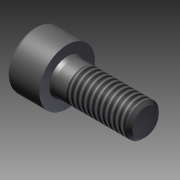
# Autodesk Inventor part: Zylinderschraube ISO 4762 - screw - M5x12-screw
Saved by Autodesk Inventor 2011 SP1 (Build 150282100, 282)
## iProperties
Created: 2016-04-05
Part Number: Zylinderschraube ISO 4762 - screw - M5x12-screw
Catalog Web Link: www.cadenas.de
Description: ISO 4762 - screw-Hexagon socket head cap screw
Vendor: MISUMI
Document SubType Name: Modeling
Designer: psAdmin
Manufacturer: MISUMI
Mass: 0.469354 g
Surface Area: 4.67275 cm^2
Volume: 0.469354 cm^3
Density: 1 g/cm^3
Category: PARTsolutions
Company: MISUMI
Title: Zylinderschraube ISO 4762 - screw - M5x12-screw
Author: Cadenas PARTsolutions
Comments: Hexagon socket head cap screw
PSOL_IDENT_0: {$CADENAS_DATA\23d-libs\misumi\metric\02_shaft_supports\screw.prj},247 {VTYP=3D},{NB=Zylinderschraub
PSOL_IDENT_1: e ISO 4762 - screw - M5x12-screw},{LINA=Zylinderschraube ISO 4762 - screw - M5x12-screw},{NN=ISO 476
PSOL_IDENT_2: 2 - screw},{DATE=22.04.2015 10:30:10},{GEOMDATE=13.12.2010 08:58:00},{VERSION=},{LINEID=490},{LINESU
PSOL_IDENT_3: BID=-1},{WBVAR=}  {NB=Zylinderschraube ISO 4762 - screw - M5x12-screw},{LINA=Zylinderschraube ISO 47
PSOL_IDENT_4: 62 - screw - M5x12-screw},{KT=DUMMY},{IDNR=},{D=5.000},{D3=4.019},{P=0.800},{L=12.000},{S=4.000},{HM=
PSOL_IDENT_5: 12.000},{DK=8.500},{DA=5.700},{DS=5.000},{E=4.580},{K=5.000},{R=0.200},{T=2.500},{V=0.500},{DW=8.030
PSOL_IDENT_6: },{W=1.900},{LF=0.600},{LG=2.400},{FORM=1.000},{NENN=M5x12-screw}
NN: ISO 4762 - screw
NT: Hexagon socket head cap screw
NB: Zylinderschraube ISO 4762 - screw - M5x12-screw
NBSYN: Zylinderschraube ISO 4762 - screw - $NENN.
LINA: Zylinderschraube ISO 4762 - screw - M5x12-screw
ROWDESC: M5x12-screw
D: 5.000
D3: 4.019
P: 0.800
L: 12.000
S: 4.000
HM: 12.000
DK: 8.500
DA: 5.700
DS: 5.000
E: 4.580
K: 5.000
R: 0.200
T: 2.500
V: 0.500
DW: 8.030
W: 1.900
LF: 0.600
LG: 2.400
FORM: 1.000
SUPPLIER: MISUMI
ARTICLENO: Zylinderschraube ISO 4762 - screw - M5x12-screw
BOMINFO: Zylinderschraube ISO 4762 - screw - M5x12-screw
CREATOR: CADENAS GmbH
Autodesk Inventor part; units mm, degrees
sketch "Skizze_2" plane through (0, 0, 0) normal (0, 0, 1) x (1, 0, 0)
  line L0 (12, 0) -> (-8, 0)
  line L1 (-0.7453, 0) -> (-1.9, 2)
  line L2 (-1.9, 2) -> (-5, 2)
  line L3 (-5, 2) -> (-5, 3.75)
  arc A0 (-4.5, 4.25) -> (-5, 3.75) centre (-4.5, 3.75) ccw
  line L4 (-4.5, 4.25) -> (0, 4.25)
  line L5 (0, 4.25) -> (0, 2.7114)
  line L6 (0, 2.7114) -> (0.5637, 2.5)
  line L7 (0.5637, 2.5) -> (11.5095, 2.5)
  line L8 (11.5095, 2.5) -> (12, 2.0095)
  line L9 (12, 2.0095) -> (12, 0)
  line L10 (12, 0) -> (-0.7453, 0)
  constraints: 22 end point, 2 point on circle, 1 centre point
revolve "Revolution1" add sketch "Skizze_2" angle 360 about axis through (12, 0, 0) along (1, 0, 0)
thread "Thread1" size "M5x0.8" class "6g" standard "ISO Metric profile" length 9.1095
sketch "Skizze_1" plane through (-1.9, 0, 0) normal (1, 0, 0) x (0, 0, -1)
  line L0 (-2, 1.1547) -> (-2, -1.1547)
  line L1 (-2, -1.1547) -> (0, -2.3094)
  line L2 (0, -2.3094) -> (2, -1.1547)
  line L3 (2, -1.1547) -> (2, 1.1547)
  line L4 (2, 1.1547) -> (0, 2.3094)
  line L5 (0, 2.3094) -> (-2, 1.1547)
  constraints: 12 end point
extrude "Extrusion1" cut sketch "Skizze_1" against normal blind 5
ref_plane "IP1_XY" through (0, 0, 0) normal (1, 0, 0) x (0, 0, -1)
ref_plane "IP1_YZ" through (0, 0, 0) normal (0, 0, -1) x (0, 1, 0)
ref_plane "IP1_ZX" through (0, 0, 0) normal (0, 1, 0) x (1, 0, 0)
ref_plane "IP2_XY" through (-5, 0, 0) normal (1, 0, 0) x (0, 0, -1)
ref_plane "IP2_YZ" through (-5, 0, 0) normal (0, 0, -1) x (0, 1, 0)
ref_plane "IP2_ZX" through (-5, 0, 0) normal (0, 1, 0) x (1, 0, 0)
ref_plane "IP3_XY" through (12, 0, 0) normal (1, 0, 0) x (0, 0, -1)
ref_plane "IP3_YZ" through (12, 0, 0) normal (0, 0, -1) x (0, 1, 0)
ref_plane "IP3_ZX" through (12, 0, 0) normal (0, 1, 0) x (1, 0, 0)
ref_plane "IP4_XY" through (0, 0, 0) normal (1, 0, 0) x (0, 0, -1)
ref_plane "IP4_YZ" through (0, 0, 0) normal (0, 0, -1) x (0, 1, 0)
ref_plane "IP4_ZX" through (0, 0, 0) normal (0, 1, 0) x (1, 0, 0)
body "Solid1"
